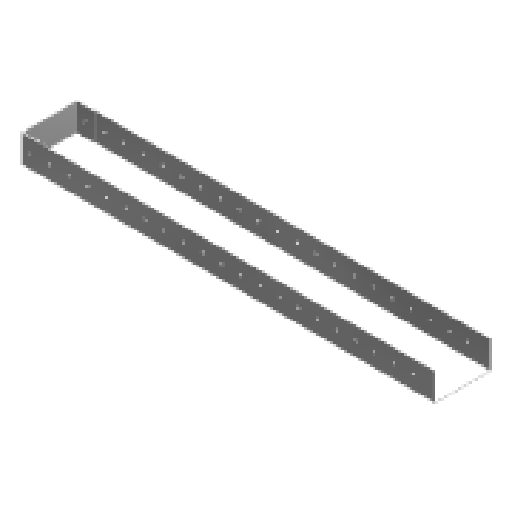
# Autodesk Inventor part: Deck
Saved by Autodesk Inventor 2025.2 (Build 292293000, 293)
## iProperties
Created: 2025-01-11
Part Number: Deck
Material: Aluminum 6061
Document SubType Name: Modeling
Designer: Authorised User
Density: 2.7 g/cm^3
Appearance: Aluminum - Flat
Author: Authorised User
Autodesk Inventor part; units mm, degrees
ref_plane "YZ Plane" through (0, 0, 0) normal (1, 0, 0) x (0, 1, 0)
ref_plane "XZ Plane" through (0, 0, 0) normal (0, 1, 0) x (-1, 0, 0)
ref_plane "XY Plane" through (0, 0, 0) normal (0, 0, 1) x (1, 0, 0)
sketch "Sketch1" plane through (0, 0, 0) normal (0, 1, 0) x (-1, 0, 0)
  line L0 (302.25, 40.25) -> (-302.25, 40.25)
  line L1 (-302.25, 40.25) -> (-302.25, -40.25)
  line L2 (-302.25, -40.25) -> (302.25, -40.25)
  line L3 (302.25, -40.25) -> (302.25, 40.25)
  line L4 (431.9097, 0) -> (-427.5376, 0) construction
  line L5 (0, 201.1267) -> (0, -116.2072) construction
  point P0 (0, 0)
  dimension "d0" = 604.5
  dimension "d1" = 80.5
  constraints: 12 end point, 3 parallel, 2 horizontal, 2 vertical, 1 perpendicular, 2 other
  measures "d0" distance of L1.end L2.end
  measures "d1" distance of L2.end L0.start
extrude "Extrusion1" add sketch "Sketch1" against normal blind 1
sketch "Sketch2" plane through (0, 0, 0) normal (0, 1, 0) x (1, 0, 0)
  line L0 (-302.25, 40.25) -> (302.25, 40.25) projected
  line L1 (-302.25, 40.25) -> (302.25, 40.25)
  line L2 (302.25, 40.25) -> (302.25, 41.25)
  line L3 (302.25, 41.25) -> (-302.25, 41.25)
  line L4 (-302.25, 41.25) -> (-302.25, 40.25)
  line L5 (302.25, -40.25) -> (-302.25, -40.25) projected
  line L6 (-302.25, -40.25) -> (302.25, -40.25)
  line L7 (302.25, -40.25) -> (302.25, -41.25)
  line L8 (302.25, -41.25) -> (-302.25, -41.25)
  line L9 (-302.25, -41.25) -> (-302.25, -40.25)
  line L10 (-302.25, -41.25) -> (-303.75, -41.25)
  line L11 (-303.75, -41.25) -> (-303.75, 42.25)
  line L12 (-303.75, 42.25) -> (-302.25, 42.25)
  line L13 (-302.25, 42.25) -> (-302.25, -41.25)
  point P0 (0, 0)
  point P1 (-300.25, 41.75)
  dimension "d4" = 1
  dimension "d5" = 604.5
  dimension "d6" = 1
  dimension "d7" = 604.5
  dimension "d8" = 1.5
  dimension "d9" = 83.5
  constraints: 24 end point, 6 parallel, 4 horizontal, 3 perpendicular
  measures "d4" distance of L3.end L0.start
  measures "d5" distance of L2.end L3.end
  measures "d6" distance of L8.end L5.end
  measures "d7" distance of L7.end L8.end
  measures "d8" distance of L8.end L10.end
  measures "d9" distance of L10.end L11.end
extrude "Extrusion2" add sketch "Sketch2" along normal blind 40 contours L4 L3 L2 L0 | L5 L7 L8 L9
sketch "Sketch3" plane through (0, 0, 0) normal (0, 1, 0) x (1, 0, 0)
  line L0 (-302.25, 41.25) -> (-302.25, 40.25) projected
  line L1 (-302.25, 41.25) -> (-302.25, 40.25) projected
  line L2 (-302.25, 41.25) -> (-302.25, 40.25) projected
  line L3 (-302.25, 41.25) -> (-302.25, 40.25) projected
  line L4 (-302.25, -40.25) -> (-302.25, 40.25) projected
  line L5 (-302.25, 40.25) -> (-302.25, -40.25) projected
  line L6 (-302.25, -40.25) -> (-302.25, -41.25) projected
  line L7 (-302.25, -40.25) -> (-302.25, -41.25) projected
  line L8 (-302.25, 40.25) -> (-302.25, -40.25) projected
  line L9 (-302.25, -40.25) -> (-302.25, 40.25) projected
  line L10 (-302.25, -40.25) -> (-302.25, -41.25) projected
  line L11 (-302.25, -40.25) -> (-302.25, -41.25) projected
  line L12 (302.25, 41.25) -> (-302.25, 41.25) projected
  line L13 (-302.25, -41.25) -> (302.25, -41.25) projected
  line L14 (302.25, -40.25) -> (-302.25, -40.25) projected
  line L15 (-302.25, 40.25) -> (302.25, 40.25) projected
  line L16 (302.25, -40.25) -> (-302.25, -40.25) projected
  line L17 (-277.25, -40.25) -> (-277.25, -39.15)
  line L18 (-277.25, -39.15) -> (-302.25, -39.15)
  line L19 (-302.25, 40.25) -> (302.25, 40.25) projected
  line L20 (-277.25, 40.25) -> (-277.25, 39.15)
  line L21 (-277.25, 39.15) -> (-302.25, 39.15)
  line L22 (-302.25, -40.25) -> (-303.35, -40.25)
  line L23 (-303.35, -40.25) -> (-303.35, 40.25)
  line L24 (-303.35, 40.25) -> (-302.25, 40.25)
  line L25 (-277.25, 40.15) -> (-303.35, 40.15)
  line L26 (-277.25, -40.15) -> (-302.25, -40.15)
  line L27 (-302.25, -40.15) -> (-303.35, -40.15)
  point P0 (0, 0)
  point P1 (-302.25, 39.15)
  dimension "d12" = 1.1
  dimension "d13" = 25
  dimension "d14" = 0.1
  dimension "d15" = 0.1
  constraints: 20 end point, 11 point on line, 8 perpendicular, 3 equal length
  measures "d12" distance of L20.start L20.end
  measures "d13" distance of L17.end L18.end
  measures "d14" distance between parallel lines of L15 L25
  measures "d15" distance between parallel lines of L22 L26
extrude "Extrusion3" add sketch "Sketch3" along normal blind 40 contours L27 L23 L25 L4 | L4 L18 L17 L26 | L4 L25 L20 L21
sketch "Sketch4" plane through (-302.25, 0, 41.25) normal (0, 0, 1) x (1, 0, 0)
  line L0 (25, 0) -> (0, 0) projected
  line L1 (25, 0) -> (25, 40) projected
  line L2 (0, 40) -> (25, 40) projected
  line L3 (0, 0) -> (0, 40) projected
  circle A0 centre (12.5, 20) radius 2
  point P0 (302.25, 0)
  point P1 (25, 20)
  point P2 (12.5, 0)
  dimension "d18" = 4
  constraints: 2 midpoint, 1 centre point, 1 horizontal alignment, 1 vertical alignment
  measures "d18" diameter of A0
extrude "Extrusion4" cut sketch "Sketch4" against normal through all contours A0
sketch "Sketch5" plane through (302.25, 0, -41.25) normal (0, 0, -1) x (-1, 0, 0)
  circle A0 centre (592, 20) radius 2 projected
  line L0 (604.5, 0) -> (0, 0) projected
  line L1 (604.5, 0) -> (604.5, 40) projected
  line L2 (0, 40) -> (604.5, 40) projected
  line L3 (0, 0) -> (0, 40) projected
  circle A1 centre (592, 20) radius 2 projected
  line L4 (604.5, 0) -> (579.5, 0) projected
  line L5 (604.5, 0) -> (604.5, 40) projected
  line L6 (579.5, 40) -> (604.5, 40) projected
  line L7 (579.5, 0) -> (579.5, 40) projected
  circle A2 centre (564, 20) radius 2
  circle A3 centre (536, 20) radius 2
  circle A4 centre (508, 20) radius 2
  circle A5 centre (480, 20) radius 2
  circle A6 centre (452, 20) radius 2
  circle A7 centre (424, 20) radius 2
  circle A8 centre (396, 20) radius 2
  circle A9 centre (368, 20) radius 2
  circle A10 centre (340, 20) radius 2
  circle A11 centre (312, 20) radius 2
  circle A12 centre (284, 20) radius 2
  circle A13 centre (256, 20) radius 2
  circle A14 centre (228, 20) radius 2
  circle A15 centre (200, 20) radius 2
  circle A16 centre (172, 20) radius 2
  circle A17 centre (144, 20) radius 2
  circle A18 centre (116, 20) radius 2
  circle A19 centre (88, 20) radius 2
  circle A20 centre (60, 20) radius 2
  circle A21 centre (32, 20) radius 2
  point P0 (302.25, 0)
  point P1 (579.5, 20)
  dimension "d21" = 4
  dimension "d22" = 15.5
  dimension "d25" = 28
  constraints: 20 centre point, 1 horizontal, 1 horizontal alignment, 1 midpoint, 38 other
  measures "d21" diameter of A2
  measures "d22" distance from line of L7 A2.centre
  measures "d25" distance of A2.centre A3.centre
extrude "Extrusion5" cut sketch "Sketch5" against normal through all contours A2 | A3 | A4 | A5 | A6 | A7 | A8 | A9 | A10 | A11 | A12 | A13 | A14 | A15 | A16 | A17 | A18 | A19 | A20 | A21
sketch "Sketch6" plane through (0, 0, 0) normal (0, 0, 1) x (1, 0, 0)
  line L0 (-277.25, 0) -> (-302.25, 0) projected
  line L1 (-302.25, 0) -> (302.25, 0) projected
  line L2 (302.25, 0) -> (-302.25, 0) projected
  line L3 (-302.25, 0) -> (-277.25, 0) projected
  line L4 (-277.25, 0) -> (-302.25, 0) projected
  line L5 (-302.25, 0) -> (-277.25, 0) projected
  line L6 (302.25, -1) -> (-302.25, -1) projected
  line L7 (-302.25, -1) -> (302.25, -1) projected
  line L8 (-299.25, -1) -> (-299.25, -2)
  line L9 (-299.25, -2) -> (-289.25, -2)
  line L10 (-289.25, -2) -> (-289.25, -11)
  line L11 (-289.25, -11) -> (-303.25, -11)
  line L12 (-303.25, -11) -> (-303.25, -12)
  line L13 (-303.25, -12) -> (-288.25, -12)
  line L14 (-288.25, -12) -> (-288.25, -1)
  point P0 (0, 0)
  point P1 (-288.25, -1)
  dimension "d32" = 1
  dimension "d33" = 3
  dimension "d34" = 1
  dimension "d35" = 1
  dimension "d36" = 11
  dimension "d37" = 10
  dimension "d38" = 15
  constraints: 14 end point, 6 perpendicular, 2 point on line, 1 vertical
  measures "d32" distance of L8.start L8.end
  measures "d33" distance from line of L6.end L8
  measures "d34" distance between parallel lines of L14 L10
  measures "d35" distance between parallel lines of L11 L13
  measures "d36" distance of L13.end L14.end
  measures "d37" distance of L8.end L9.end
  measures "d38" distance of L12.end L13.end
extrude "Extrusion6" add sketch "Sketch6" along normal mid plane 25
chamfer "Chamfer1" distance 5 angle 45 2 edges at (-303.25, -11.5, 12.5) (-303.25, -11.5, -12.5)
equation "\"d34\" = d32"
equation "\"d35\" = d32"
body "Solid1"
